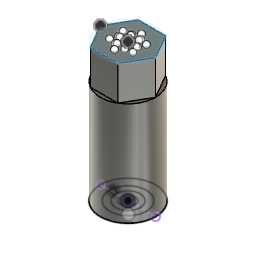
Aquazepp_Schraube v4 (Autodesk Fusion 360 design; units mm, degrees)
Autodesk Fusion 360 part; units mm, degrees
sketch "Skizze1" plane through (0, 0, 0) normal (0, 0, 1) x (1, 0, 0)
  circle A0 centre (0, 0) radius 8
  circle A1 centre (0, 0) radius 2
  circle A2 centre (0, 0) radius 3.5
  circle A3 centre (0, 0) radius 5.3
  dimension "d1" = 16
  dimension "d2" = 4
  dimension "d5" = 7
  dimension "d7" = 1.8
  constraint coincident A0.centre A1.centre
  constraint concentric A0 A1
  constraint concentric A0 A2
  measures "d1" diameter of A0
  measures "d2" diameter of A1
  measures "d5" diameter of A2
extrude "Extrusion1" add sketch "Skizze1" along normal blind 40 contours A0 | A2 | A3
extrude "Extrusion2" [suppressed]
sketch "Skizze2" plane through (0, 0, 40) normal (0, 0, 1) x (-1, 0, 0)
  circle A0 centre (0, 0) radius 2
  circle A1 centre (0, 0) radius 8
  line L0 (8, 0) -> (4, 6.9282)
  line L1 (4, 6.9282) -> (-4, 6.9282)
  line L2 (-4, 6.9282) -> (-8, 0)
  line L3 (-8, 0) -> (-4, -6.9282)
  line L4 (-4, -6.9282) -> (4, -6.9282)
  line L5 (4, -6.9282) -> (8, 0)
  constraint coincident A1 L0.start
  constraint coincident A0.centre A1.centre
extrude "Extrusion3" cut sketch "Skizze2" against normal blind 10 contours A1 L0 | A1 L5 | A1 L1 | A1 L4 | A1 L2 | A1 L3
sketch "Skizze3" plane through (0, 0, 40) normal (0, 0, 1) x (-1, 0, 0)
  line L0 (8, 0) -> (4, 6.9282)
  line L1 (4, 6.9282) -> (-4, 6.9282)
  line L2 (-4, 6.9282) -> (-8, 0)
  line L3 (-8, 0) -> (-4, -6.9282)
  line L4 (-4, -6.9282) -> (4, -6.9282)
  line L5 (4, -6.9282) -> (8, 0)
  circle A0 centre (0, 0) radius 2
  arc A1 (1.3826, -2.3693) -> (1.5865, -2.0034) centre (1.1752, -2.0139) ccw
  arc A2 (1.3826, -2.3693) -> (1.5865, -2.0034) centre (1.1752, -2.0139) ccw
  arc A3 (1.5865, 2.0034) -> (2.5283, 0.3723) centre (3.3901, 1.9573) ccw
  arc A4 (-1.3826, 2.3693) -> (-1.5865, 2.0034) centre (-1.1752, 2.0139) ccw
  arc A5 (1.3606, 2.382) -> (0.9417, 2.3757) centre (1.1565, 2.0247) ccw
  arc A6 (2.5283, -0.3723) -> (2.7432, -0.0127) centre (2.3317, -0.0108) ccw
  arc A7 (1.3826, 2.3693) -> (1.3606, 2.382) centre (0, 0) ccw
  arc A8 (-1.5865, -2.0034) -> (-1.3826, -2.3693) centre (-1.1752, -2.0139) ccw
  arc A9 (-1.3826, -2.3693) -> (-1.3606, -2.382) centre (0, 0) ccw
  arc A10 (-1.5865, -2.0034) -> (-2.5283, -0.3723) centre (-3.3901, -1.9573) ccw
  arc A11 (-2.5283, 0.3723) -> (-1.5865, 2.0034) centre (-3.3901, 1.9573) ccw
  arc A12 (2.5283, -0.3723) -> (2.7432, -0.0127) centre (2.3317, -0.0108) ccw
  arc A13 (-2.5283, 0.3723) -> (-2.7432, 0.0127) centre (-2.3317, 0.0108) ccw
  arc A14 (-0.9417, 2.3757) -> (-1.3606, 2.382) centre (-1.1565, 2.0247) ccw
  arc A15 (-2.7432, -0.0127) -> (-2.5283, -0.3723) centre (-2.3317, -0.0108) ccw
  arc A16 (2.7432, 0.0127) -> (2.5283, 0.3723) centre (2.3317, 0.0108) ccw
  arc A17 (1.5865, 2.0034) -> (1.3826, 2.3693) centre (1.1752, 2.0139) ccw
  arc A18 (1.5865, 2.0034) -> (2.5283, 0.3723) centre (3.3901, 1.9573) ccw
  arc A19 (-1.5865, -2.0034) -> (-1.3826, -2.3693) centre (-1.1752, -2.0139) ccw
  arc A20 (0.9417, -2.3757) -> (-0.9417, -2.3757) centre (0, -3.9145) ccw
  arc A21 (2.7432, -0.0127) -> (2.7432, 0.0127) centre (0, 0) ccw
  arc A22 (-2.7432, 0.0127) -> (-2.7432, -0.0127) centre (0, 0) ccw
  arc A23 (-1.3826, 2.3693) -> (-1.5865, 2.0034) centre (-1.1752, 2.0139) ccw
  arc A24 (-1.3606, -2.382) -> (-0.9417, -2.3757) centre (-1.1565, -2.0247) ccw
  arc A25 (0.9417, -2.3757) -> (-0.9417, -2.3757) centre (0, -3.9145) ccw
  arc A26 (-1.3606, 2.382) -> (-1.3826, 2.3693) centre (0, 0) ccw
  arc A27 (1.5865, 2.0034) -> (1.3826, 2.3693) centre (1.1752, 2.0139) ccw
  arc A28 (-1.3606, -2.382) -> (-0.9417, -2.3757) centre (-1.1565, -2.0247) ccw
  arc A29 (-0.9417, 2.3757) -> (0.9417, 2.3757) centre (0, 3.9145) ccw
  arc A30 (2.7432, 0.0127) -> (2.5283, 0.3723) centre (2.3317, 0.0108) ccw
  arc A31 (-2.7432, -0.0127) -> (-2.5283, -0.3723) centre (-2.3317, -0.0108) ccw
  arc A32 (-0.9417, 2.3757) -> (-1.3606, 2.382) centre (-1.1565, 2.0247) ccw
  arc A33 (2.5283, -0.3723) -> (1.5865, -2.0034) centre (3.3901, -1.9573) ccw
  arc A34 (-1.5865, -2.0034) -> (-2.5283, -0.3723) centre (-3.3901, -1.9573) ccw
  arc A35 (-0.9417, 2.3757) -> (0.9417, 2.3757) centre (0, 3.9145) ccw
  arc A36 (1.3606, -2.382) -> (1.3826, -2.3693) centre (0, 0) ccw
  arc A37 (-2.5283, 0.3723) -> (-2.7432, 0.0127) centre (-2.3317, 0.0108) ccw
  arc A38 (-2.5283, 0.3723) -> (-1.5865, 2.0034) centre (-3.3901, 1.9573) ccw
  arc A39 (1.3606, 2.382) -> (0.9417, 2.3757) centre (1.1565, 2.0247) ccw
  arc A40 (2.5283, -0.3723) -> (1.5865, -2.0034) centre (3.3901, -1.9573) ccw
  arc A41 (0.9417, -2.3757) -> (1.3606, -2.382) centre (1.1565, -2.0247) ccw
  arc A42 (0.9417, -2.3757) -> (1.3606, -2.382) centre (1.1565, -2.0247) ccw
extrude "Extrusion4" cut sketch "Skizze3" against normal blind 6 contours A1 A2 A3 A4 A5 A6 A7 A8 A9 A10 A11 A12 A13 A14 A15 A16 A17 A18 A19 A20 A21 A22 A23 A24 A25 A26 A27 A28 A29 A30 A31 A32 A33 A34 A35 A36 A37 A38 A39 A40 A41 A42
sketch "Skizze4" plane through (0, 0, 0) normal (0, 1, 0) x (1, 0, 0)
  circle A0 centre (-4.3, -0.45) radius 0.86
  line L0 (0, 0) -> (0, 3.4196) construction
  line L1 (-8, 0) -> (8, 0)
  dimension "d14" = 1.72
  dimension "d15" = 4.3
  dimension "d17" = 0.45
  constraint coincident L0.start origin
  constraint vertical L0
  measures "d14" diameter of A0
  measures "d15" distance of A0.centre L0
  measures "d17" distance of A0.centre L1
revolve "Drehen1" cut sketch "Skizze4" angle 360 about axis through (0, 0, 0) along (0, 0, -1)
thread "Gewinde1" "ISO Metric profile 5.0 M5x0.8 6H" major diameter 5.12 minor diameter 4.234 pitch 0.8 angle 60 modelled right hand crest width 0.2219 on face at (1.9901, 0.1991, 22.6667) crest through (2.117, 0, 0.2)
equation "d15 = ( 8.6 / 2 ) * 1 mm"
named bodies: "Aquazepp_Schraube"
